011 (Autodesk Fusion 360 design; units mm, degrees)
Autodesk Fusion 360 part; units mm, degrees
sketch "Esquisse1" plane through (0, 0, 0) normal (0, 0, 1) x (1, 0, 0)
  circle A0 centre (0, 0) radius 24
  dimension "d1" = 48
  constraint coincident A0.centre origin
  measures "d1" diameter of A0
extrude "Extrusion1" add sketch "Esquisse1" along normal blind 10
sketch "Esquisse2" plane through (0, 0, 10) normal (0, 0, 1) x (-1, 0, 0)
  circle A0 centre (0, 0) radius 24
  circle A1 centre (0, 0) radius 4.5
  dimension "d4" = 9
  constraint coincident A0.centre A1.centre
  measures "d4" diameter of A1
extrude "Extrusion2" cut sketch "Esquisse2" against normal blind 3 contours A1
sketch "Esquisse3" plane through (0, 0, 10) normal (0, 0, 1) x (-1, 0, 0)
  circle A0 centre (0, 0) radius 4.5
  circle A1 centre (0, 0) radius 24
  circle A2 centre (20, 0) radius 3
  dimension "d7" = 20
  dimension "d17" = 6
  measures "d7" distance of A0.centre A2.centre
  measures "d17" diameter of A2
extrude "Extrusion3" add sketch "Esquisse3" along normal blind 15 contours A2
mirror "Symétrie miroir1" about plane through (0, 0, 0) normal (1, 0, 0) of "Extrusion3"
sketch "Esquisse4" plane through (0, 0, 25) normal (0, 0, 1) x (-1, 0, 0)
  circle A0 centre (20, 0) radius 3
  circle A1 centre (20, 0) radius 2.25
  dimension "d12" = 4.5
  constraint concentric A0 A1
  measures "d12" diameter of A1
extrude "Extrusion4" cut sketch "Esquisse4" against normal blind 36 contours A1
mirror "Symétrie miroir2" about plane through (0, 0, 0) normal (1, 0, 0) of "Extrusion4"
sketch "Esquisse5" plane through (0, 0, 10) normal (0, 0, 1) x (-1, 0, 0)
  circle A0 centre (-20, 0) radius 3
  circle A1 centre (20, 0) radius 3
  circle A2 centre (0, 0) radius 4.5
  circle A3 centre (0, 0) radius 24
sketch "Esquisse6" plane through (0, 0, 10) normal (0, 0, 1) x (-1, 0, 0)
  line L0 (29.6799, -30) -> (-29.6799, -30)
  line L1 (-29.6799, -30) -> (-29.6799, -15)
  line L2 (-29.6799, -15) -> (29.6799, -15)
  line L3 (29.6799, -15) -> (29.6799, -30)
  line L4 (0, -1.75) -> (0, -22.5)
  line L5 (-20, 0) -> (-2.5, 0)
  dimension "d18" = 15
  dimension "d19" = 15
  constraint horizontal L0
  constraint vertical L1
  constraint horizontal L2
  constraint vertical L3
  constraint symmetric L1 L3 L4
  measures "d18" distance of L2 L5
  measures "d19" distance of L0.start L2.end
extrude "Extrusion5" cut sketch "Esquisse6" against normal blind 25
mirror "Symétrie miroir3" about plane through (0, 0, 0) normal (0, 1, 0) of "Extrusion5"
